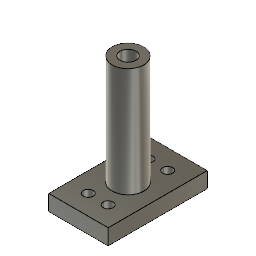
rod_support (Autodesk Fusion 360 design; units mm, degrees)
Autodesk Fusion 360 part; units mm, degrees
note: some values were not read from the file. Chosen so that the rebuilt part matches the saved one: which face or edge a step refers to.
sketch "Sketch1" plane through (0, 0, 0) normal (0, 0, 1) x (1, 0, 0)
  line L0 (0, 0) -> (30, 0)
  line L1 (30, 0) -> (30, 50)
  line L2 (30, 50) -> (0, 50)
  line L3 (0, 50) -> (0, 0)
  line L4 (15, 50) -> (15, 0)
  line L5 (0, 25) -> (30, 25)
  dimension "d16" = 15
  constraint horizontal L0
  constraint vertical L1
  constraint horizontal L2
  constraint vertical L3
  constraint coincident L0.start L3.end
  constraint midpoint L2 L4.start
  constraint midpoint L0 L4.end
  constraint midpoint L3 L5.start
  constraint midpoint L1 L5.end
  measures "d16" distance of L3 L4
extrude "Extrude1" add sketch "Sketch1" along normal blind 8
sketch "Sketch6" plane through (0, 0, 8) normal (0, 0, 1) x (-1, 0, 0)
  line L0 (0, -50) -> (0, 0)
  line L1 (0, 0) -> (-30, 0)
  line L2 (-30, 0) -> (-30, -50)
  line L3 (-30, -50) -> (0, -50)
  line L4 (-15, -50) -> (-15, 0)
  line L5 (0, -25) -> (-30, -25)
  circle A0 centre (-15, -25) radius 8
  circle A1 centre (-15, -25) radius 4
  dimension "d17" = 16
  dimension "d18" = 8
  constraint midpoint L3 L4.start
  constraint midpoint L1 L4.end
  constraint midpoint L0 L5.start
  constraint midpoint L2 L5.end
  constraint midpoint L5 A0.centre
  constraint concentric A0 A1
  measures "d17" diameter of A0
  measures "d18" diameter of A1
extrude "Extrude5" add sketch "Sketch6" along normal blind 30 contours L4 L5 A0 A1 | L4 L5 A0 A1 | L4 L5 A0 A1 | L4 L5 A0 A1
sketch "Sketch7" plane through (0, 0, 8) normal (0, 0, 1) x (-1, 0, 0)
  line L0 (0, -50) -> (0, 0)
  line L1 (0, 0) -> (-30, 0)
  line L2 (-30, 0) -> (-30, -50)
  line L3 (-30, -50) -> (0, -50)
  circle A0 centre (-15, -25) radius 8
  circle A1 centre (-10, -40) radius 2.5
  circle A2 centre (-20, -40) radius 2.5
  circle A3 centre (-10, -5) radius 2.5
  circle A4 centre (-20, -10) radius 2.5
  circle A5 centre (-10, -10) radius 2.5
  dimension "d21" = 5
  dimension "d22" = 5
  dimension "d23" = 10
  dimension "d24" = 10
  dimension "d25" = 5
  dimension "d26" = 5
  dimension "d27" = 5
  measures "d21" diameter of A1
  measures "d22" diameter of A2
  measures "d23" distance of L0 A1.centre
  measures "d24" distance of L2 A2.centre
  measures "d25" diameter of A3
  measures "d26" diameter of A4
  measures "d27" diameter of A5
extrude "Extrude6" cut sketch "Sketch7" against normal blind 10 contours A1 | A2 | A5 | A4
sketch "Sketch8" plane through (0, 0, 38) normal (0, 0, 1) x (-1, 0, 0)
  circle A0 centre (-15, -25) radius 4
  circle A1 centre (-15, -25) radius 8
extrude "Extrude7" add sketch "Sketch8" along normal blind 10
sketch "Sketch12" plane through (0, 0, 0) normal (0, 1, 0) x (1, 0, 0)
extrude "Extrude9" add 1 faces at (8.378, 25.5962, 48) along direction (0, 0, 1) blind 15
extrude "Extrude10" add 1 faces at (14.1687, 26.0424, 8) along direction (0, 0, 1) blind 15
sketch "Sketch9" plane through (0, 0, 48) normal (0, 0, 1) x (-1, 0, 0)
  circle A0 centre (-15, -25) radius 4
  circle A1 centre (-15, -25) radius 8
sketch "Sketch10" plane through (0, 0, 0) normal (1, 0, 0) x (0, 1, 0)
